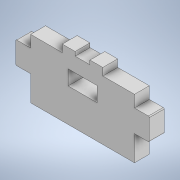
# Autodesk Inventor part: extra_switch_support
Saved by Autodesk Inventor 2020 (Build 240168000, 168)
## iProperties
Created: 2019-07-10
Part Number: extra_switch_support
Material: Générique
Document SubType Name: Modeling
Designer: Thibault
Density: 1 g/cm^3
Appearance: Par défaut
Mass: 0.1094 g
Surface Area: 2.51573 cm^2
Volume: 0.1094 cm^3
d18: 2.000 mm
d19: 2.000 mm
d20: 2.000 mm
d21: 2.000 mm
d22: 2.000 mm
d23: 15.00 deg
d24: 15.00 deg
d25: 0.00 deg
d26: 2.000 mm
d27: 2.000 mm
d28: 4.000 mm
d29: 345.00 deg
d30: 330.00 deg
Author: Thibault
Autodesk Inventor part; units mm, degrees
ref_plane "YZ Plane" through (0, 0, 0) normal (1, 0, 0) x (0, 1, 0)
ref_plane "XZ Plane" through (0, 0, 0) normal (0, 1, 0) x (-1, 0, 0)
ref_plane "XY Plane" through (0, 0, 0) normal (0, 0, 1) x (1, 0, 0)
sketch "Unit" plane through (0, 0, 0) normal (0, 0, 1) x (1, 0, 0)
  line L0 (17.4453, 22.2497) -> (21.7153, 22.2497)
  line L1 (21.7153, 22.2497) -> (21.7153, 23.2497)
  line L2 (21.7153, 23.2497) -> (23.4453, 23.2497)
  line L3 (21.7153, 23.2497) -> (21.7153, 24.9797) construction
  line L4 (23.4453, 23.2497) -> (23.4453, 22.6997)
  line L5 (23.4453, 22.6997) -> (25.4453, 22.6997)
  line L6 (25.4453, 22.6997) -> (25.4453, 23.2497)
  line L7 (25.4453, 23.2497) -> (27.1753, 23.2497)
  line L8 (27.1753, 23.2497) -> (27.1753, 22.2497)
  line L9 (27.1753, 22.2497) -> (31.4453, 22.2497)
  line L10 (26.3953, 20.7497) -> (22.4953, 20.7497)
  line L11 (22.4953, 20.7497) -> (22.4953, 18.7497)
  line L12 (22.4953, 18.7497) -> (26.3953, 18.7497)
  line L13 (26.3953, 18.7497) -> (26.3953, 20.7497)
  line L14 (26.3953, 20.7497) -> (22.4953, 18.7497) construction
  line L15 (22.4953, 20.7497) -> (26.3953, 18.7497) construction
  point P0 (20.0288, 26.7181)
  point P1 (24.4453, 19.7497)
  dimension "d17" = 2
  dimension "d31" = 110
  dimension "d32" = 0
  dimension "d33" = 2
  dimension "d34" = 20
  dimension "d35" = 20
  dimension "d36" = 1.5
  dimension "d37" = 20.3526
  dimension "d2" = 1
  dimension "d3" = 1.73
  dimension "d4" = 0.55
  dimension "d5" = 2
  dimension "d6" = 1.73
  dimension "d7" = 1
  dimension "d12" = 3.9
  dimension "d13" = 2
  dimension "d14" = 1.5
  dimension "d40" = 14
  measures "d2" distance of L0.end L1.end
  measures "d3" distance of L1.end L2.end
  measures "d4" distance of L2.end L4.end
  measures "d5" distance of L4.end L5.end
  measures "d6" distance of L6.end L7.end
  measures "d7" distance of L7.end L8.end
  measures "d12" distance of L12.end L11.end
  measures "d13" distance of L11.end L10.end
  measures "d14" vertical distance of L0.end L10.end
  measures "d40" distance of L9.end L0.start
sketch "Anchor" plane through (0, 0, 0) normal (0, 0, 1) x (1, 0, 0)
  line L0 (1.6, 0) -> (1.6, 1.875)
  line L1 (1.6, 0) -> (2.6, 0) construction
  line L2 (1.725, 2) -> (4.475, 2)
  line L3 (4.6, 1.875) -> (4.6, 0)
  line L4 (4.6, 2) -> (6.6, 2) construction
  line L5 (0, 0) -> (1.6, 0)
  line L6 (4.6, 0) -> (6.2, 0)
  arc A0 (1.725, 2) -> (1.6, 1.875) centre (1.725, 1.875) ccw
  arc A1 (4.6, 1.875) -> (4.475, 2) centre (4.475, 1.875) ccw
  point P0 (9.1321, -0.6227)
  point P1 (1.6, 2)
  dimension "d69" = 15
  dimension "d45" = 1.6
  dimension "d46" = 2
  dimension "d47" = 3
  dimension "d48" = 2
  dimension "d60" = 1.6
  dimension "d67" = 0.125
  measures "d45" distance of point (0, 0) L0.start
  measures "d46" distance of L0.start point (1.6, 2)
  measures "d47" distance of point (1.6, 2) L4.start
  measures "d48" distance of L3.end L4.start
  measures "d60" distance of L3.end point (6.2, 0)
  measures "d67" radius of A0
sketch "Esquisse2" plane through (0, 0, 0) normal (0, 0, 1) x (1, 0, 0)
  line L0 (-10.7803, -15.7535) -> (3.2197, -15.7535)
  line L1 (-10.7803, -13.9535) -> (-10.7803, -15.7535)
  line L2 (3.2197, -13.9535) -> (3.2197, -15.7535)
  line L3 (-10.7803, -12.3535) -> (-12.6553, -12.3535)
  line L4 (-10.7803, -12.3535) -> (-10.7803, -11.3535) construction
  line L5 (-12.7803, -12.2285) -> (-12.7803, -9.4785)
  line L6 (-12.6553, -9.3535) -> (-10.7803, -9.3535)
  line L7 (-12.7803, -9.3535) -> (-12.7803, -7.3535) construction
  line L8 (-10.7803, -13.9535) -> (-10.7803, -12.3535)
  line L9 (-10.7803, -9.3535) -> (-10.7803, -7.7535)
  arc A0 (-12.7803, -12.2285) -> (-12.6553, -12.3535) centre (-12.6553, -12.2285) ccw
  arc A1 (-12.6553, -9.3535) -> (-12.7803, -9.4785) centre (-12.6553, -9.4785) ccw
  line L10 (3.2197, -9.3535) -> (5.0947, -9.3535)
  line L11 (3.2197, -9.3535) -> (3.2197, -10.3535) construction
  line L12 (5.2197, -9.4785) -> (5.2197, -12.2285)
  line L13 (5.0947, -12.3535) -> (3.2197, -12.3535)
  line L14 (5.2197, -12.3535) -> (5.2197, -14.3535) construction
  line L15 (3.2197, -7.7535) -> (3.2197, -9.3535)
  line L16 (3.2197, -12.3535) -> (3.2197, -13.9535)
  arc A2 (5.2197, -9.4785) -> (5.0947, -9.3535) centre (5.0947, -9.4785) ccw
  arc A3 (5.0947, -12.3535) -> (5.2197, -12.2285) centre (5.0947, -12.2285) ccw
  line L17 (-10.7803, -7.7535) -> (-6.5103, -7.7535)
  line L18 (-6.5103, -7.7535) -> (-6.5103, -6.7535)
  line L19 (-6.5103, -6.7535) -> (-4.7803, -6.7535)
  line L20 (-6.5103, -6.7535) -> (-6.5103, -5.0235) construction
  line L21 (-4.7803, -6.7535) -> (-4.7803, -7.3035)
  line L22 (-4.7803, -7.3035) -> (-2.7803, -7.3035)
  line L23 (-2.7803, -7.3035) -> (-2.7803, -6.7535)
  line L24 (-2.7803, -6.7535) -> (-1.0503, -6.7535)
  line L25 (-1.0503, -6.7535) -> (-1.0503, -7.7535)
  line L26 (-1.0503, -7.7535) -> (3.2197, -7.7535)
  line L27 (-1.8303, -9.2535) -> (-5.7303, -9.2535)
  line L28 (-5.7303, -9.2535) -> (-5.7303, -11.2535)
  line L29 (-5.7303, -11.2535) -> (-1.8303, -11.2535)
  line L30 (-1.8303, -11.2535) -> (-1.8303, -9.2535)
  line L31 (-1.8303, -9.2535) -> (-5.7303, -11.2535) construction
  line L32 (-5.7303, -9.2535) -> (-1.8303, -11.2535) construction
  point P0 (0, 0)
  point P1 (3.2197, -7.7535)
  point P2 (-10.7803, -10.7535)
  point P3 (3.2197, -10.7535)
  dimension "d89" = 8
  constraints: 6 end point, 2 vertical, 1 horizontal, 2 other
extrude "Extrusion1" add sketch "Esquisse2" along normal blind 2
equation "\"d35\" = d34"
equation "\"d6\" = d3"
equation "\"d7\" = d2"
equation "\"d13\" = sheet_thickness"
equation "\"d45\" = safe_distance"
equation "\"d46\" = sheet_thickness"
equation "\"d47\" = 1.5 * sheet_thickness"
equation "\"d48\" = sheet_thickness"
equation "\"d89\" = 4 * sheet_thickness"
equation "\"d71\" = sheet_thickness"
equation "\"d60\" = safe_distance"
equation "\"sheet_thickness\" = 2"
equation "\"safe_distance\" = 1.6"
